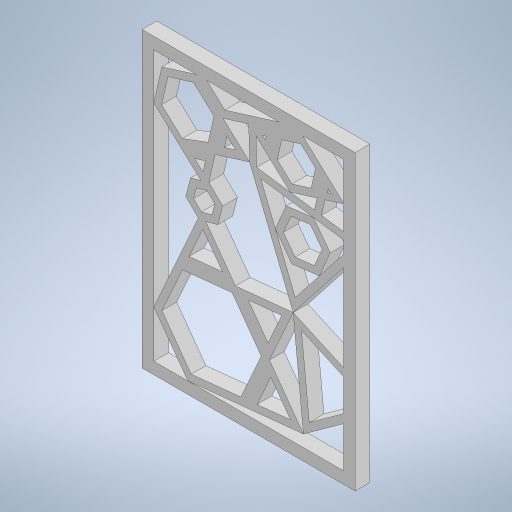
# Autodesk Inventor part: стена
Saved by Autodesk Inventor 2023.1 (Build 271208000, 208)
## iProperties
Created: 2025-12-15
Part Number: стена
Material: Типовые
Document SubType Name: Modeling
Designer: DELL
Density: 1 g/cm^3
Appearance: По умолчанию
Author: DELL
Autodesk Inventor part; units mm, degrees
ref_plane "YZ Plane" through (0, 0, 0) normal (1, 0, 0) x (0, 1, 0)
ref_plane "XZ Plane" through (0, 0, 0) normal (0, 1, 0) x (-1, 0, 0)
ref_plane "XY Plane" through (0, 0, 0) normal (0, 0, 1) x (1, 0, 0)
sketch "Эскиз1" plane through (0, 0, 0) normal (0, 0, 1) x (1, 0, 0)
  line L0 (-18.1641, 25.0477) -> (18.0359, 25.0477)
  line L1 (18.0359, 25.0477) -> (18.0359, -24.7523)
  line L2 (18.0359, -24.7523) -> (-18.1641, -24.7523)
  line L3 (-18.1641, -24.7523) -> (-18.1641, 25.0477)
  line L4 (16.0359, -22.7523) -> (16.0359, 23.0477)
  line L5 (16.0359, 23.0477) -> (-16.1641, 23.0477)
  line L6 (-16.1641, 23.0477) -> (-16.1641, -22.7523)
  line L7 (-16.1641, -22.7523) -> (16.0359, -22.7523)
  line L8 (-10.3906, -22.7523) -> (-16.1641, -14.7523)
  line L9 (-16.1641, -14.7523) -> (-12.1226, -5.7523)
  line L10 (-12.1226, -5.7523) -> (-2.3077, -4.7523)
  line L11 (-2.3077, -4.7523) -> (3.4658, -12.7523)
  line L12 (3.4658, -12.7523) -> (-0.5756, -21.7523)
  line L13 (-0.5756, -21.7523) -> (-10.3906, -22.7523)
  line L14 (-1.3865, -20.6287) -> (2.0873, -12.8928)
  line L15 (2.0873, -12.8928) -> (-2.8753, -6.0164)
  line L16 (-2.8753, -6.0164) -> (-11.3118, -6.8759)
  line L17 (-11.3118, -6.8759) -> (-14.7856, -14.6119)
  line L18 (-14.7856, -14.6119) -> (-9.823, -21.4883)
  line L19 (-9.823, -21.4883) -> (-1.3865, -20.6287)
  line L20 (-0.5756, -21.7523) -> (9.2393, -20.7523)
  line L21 (9.2393, -20.7523) -> (3.4658, -12.7523)
  line L22 (7.0499, -19.7692) -> (1.3705, -20.3478)
  line L23 (3.7091, -15.14) -> (1.3705, -20.3478)
  line L24 (3.7091, -15.14) -> (7.0499, -19.7692)
  line L25 (-12.1226, -5.7523) -> (-8.0812, 3.2477)
  line L26 (-8.0812, 3.2477) -> (-2.3077, -4.7523)
  line L27 (-2.3077, -4.7523) -> (-12.1226, -5.7523)
  line L28 (-10.1765, -4.3478) -> (-4.4971, -3.7692)
  line L29 (-4.4971, -3.7692) -> (-7.8379, 0.86)
  line L30 (-7.8379, 0.86) -> (-10.1765, -4.3478)
  line L31 (3.4658, -12.7523) -> (-2.3077, -4.7523)
  line L32 (-2.3077, -4.7523) -> (7.5073, -3.7523)
  line L33 (7.5073, -3.7523) -> (3.4658, -12.7523)
  line L34 (-0.1183, -5.7355) -> (5.5611, -5.1568)
  line L35 (5.5611, -5.1568) -> (3.2226, -10.3647)
  line L36 (-0.1183, -5.7355) -> (3.2226, -10.3647)
  line L37 (-11.6503, 11.0477) -> (-16.1641, 15.2295)
  line L38 (-16.1641, 15.2295) -> (-14.7994, 21.2295)
  line L39 (-14.7994, 21.2295) -> (-8.9209, 23.0477)
  line L40 (-8.9209, 23.0477) -> (-4.4071, 18.8658)
  line L41 (-4.4071, 18.8658) -> (-5.7718, 12.8658)
  line L42 (-7.1851, 12.4287) -> (-10.4106, 11.4311)
  line L43 (-9.4452, 21.6294) -> (-13.783, 20.2878)
  line L44 (-13.783, 20.2878) -> (-14.8403, 15.6389)
  line L45 (-14.8403, 15.6389) -> (-11.3471, 12.4027)
  line L46 (-11.3471, 12.4027) -> (-6.9303, 14.0695)
  line L47 (-6.9303, 14.0695) -> (-5.9478, 18.3893)
  line L48 (-5.9478, 18.3893) -> (-9.4452, 21.6294)
  line L49 (-5.7718, 12.8658) -> (-7.1365, 6.8658)
  line L50 (-7.1365, 6.8658) -> (-11.6503, 11.0477)
  line L51 (-10.4106, 11.4311) -> (-7.1851, 12.4287)
  line L52 (-7.4029, 11.1053) -> (-7.8262, 9.2438)
  line L53 (-7.8262, 9.2438) -> (-9.2237, 10.5421)
  line L54 (-5.7718, 12.8658) -> (-4.4071, 18.8658)
  line L55 (-4.4071, 18.8658) -> (0.1067, 14.684)
  line L56 (0.1067, 14.684) -> (-5.7718, 12.8658)
  line L57 (-2.2854, 15.2681) -> (-4.1564, 14.6894)
  line L58 (-3.7221, 16.5991) -> (-2.2854, 15.2681)
  line L59 (-3.7221, 16.5991) -> (-4.1564, 14.6894)
  line L60 (-7.4029, 11.1053) -> (-9.2237, 10.5421)
  line L61 (-5.7718, 12.8658) -> (-7.1851, 12.4287)
  line L62 (-10.4106, 11.4311) -> (-11.6503, 11.0477)
  line L63 (7.5073, -3.7523) -> (0.1067, 14.684)
  line L64 (16.0359, 7.1134) -> (7.5073, -3.7523)
  line L65 (16.0359, 9.0569) -> (7.8466, -1.3764)
  line L66 (1.9946, 13.2022) -> (16.0359, 11.1966)
  line L67 (7.8466, -1.3764) -> (1.9946, 13.2022)
  line L68 (0.1067, 14.684) -> (16.0359, 12.4088)
  line L69 (11.9413, 3.8402) -> (7.2772, 3.2858)
  line L70 (7.2772, 3.2858) -> (4.465, 7.0478)
  line L71 (4.465, 7.0478) -> (6.3169, 11.3642)
  line L72 (6.3169, 11.3642) -> (10.981, 11.9186)
  line L73 (10.981, 11.9186) -> (13.7931, 8.1566)
  line L74 (13.7931, 8.1566) -> (11.9413, 3.8402)
  line L75 (7.8235, 4.5592) -> (11.1116, 4.9501)
  line L76 (11.1116, 4.9501) -> (12.4172, 7.9931)
  line L77 (12.4172, 7.9931) -> (10.4346, 10.6452)
  line L78 (10.4346, 10.6452) -> (7.1465, 10.2543)
  line L79 (7.1465, 10.2543) -> (5.841, 7.2113)
  line L80 (5.841, 7.2113) -> (7.8235, 4.5592)
  line L81 (7.5073, -3.7523) -> (9.2393, -20.7523)
  line L82 (9.2393, -20.7523) -> (16.0359, -15.8473)
  line L83 (7.5073, -3.7523) -> (16.0359, -7.5821)
  line L84 (8.9118, -5.6985) -> (16.0359, -8.8976)
  line L85 (10.2225, -18.5629) -> (16.0359, -14.3675)
  line L86 (8.9118, -5.6985) -> (10.2225, -18.5629)
  line L87 (-4.4071, 18.8658) -> (9.1135, 23.0477)
  line L88 (-4.0998, 20.217) -> (5.0524, 23.0477)
  line L89 (-4.0998, 20.217) -> (-7.1552, 23.0477)
  line L90 (6.9877, 13.7011) -> (3.472, 16.9583)
  line L91 (3.472, 16.9583) -> (4.5349, 21.6315)
  line L92 (4.5349, 21.6315) -> (9.1135, 23.0477)
  line L93 (9.1135, 23.0477) -> (12.6293, 19.7905)
  line L94 (12.6293, 19.7905) -> (11.5663, 15.1173)
  line L95 (11.5663, 15.1173) -> (6.9877, 13.7011)
  line L96 (11.3055, 19.3811) -> (8.8062, 21.6965)
  line L97 (8.8062, 21.6965) -> (5.5514, 20.6898)
  line L98 (5.5514, 20.6898) -> (4.7958, 17.3677)
  line L99 (4.7958, 17.3677) -> (7.295, 15.0523)
  line L100 (7.295, 15.0523) -> (10.5499, 16.059)
  line L101 (10.5499, 16.059) -> (11.3055, 19.3811)
  line L102 (11.5663, 15.1173) -> (12.6293, 19.7905)
  line L103 (12.6293, 19.7905) -> (16.0359, 16.6344)
  line L104 (16.145, 16.5334) -> (16.0359, 16.4997) construction
  line L105 (16.0359, 16.6344) -> (16.145, 16.5334) construction
  line L106 (13.4535, 17.3911) -> (13.9482, 16.9327)
  line L107 (13.9482, 16.9327) -> (13.3039, 16.7334)
  line L108 (13.4535, 17.3911) -> (13.3039, 16.7334)
  line L109 (16.0359, 16.4997) -> (11.5663, 15.1173)
  line L110 (12.6293, 19.7905) -> (11.1103, 13.1123)
  line L111 (4.5349, 21.6315) -> (3.472, 16.9583)
  line L112 (3.472, 16.9583) -> (-0.0437, 20.2154)
  line L113 (-0.0437, 20.2154) -> (4.5349, 21.6315)
  line L114 (6.9877, 13.7011) -> (11.1103, 13.1123)
  line L115 (-0.0437, 20.2154) -> (0.1067, 14.684)
  line L116 (1.1878, 19.0745) -> (1.3118, 14.5119)
  line L117 (2.2965, 19.6831) -> (2.9039, 19.871)
  line L118 (2.7629, 19.2511) -> (2.2965, 19.6831)
  line L119 (2.7629, 19.2511) -> (2.9039, 19.871)
  line L120 (12.3023, 12.942) -> (12.8901, 15.5267)
  line L121 (-8.0812, 3.2477) -> (-9.4117, 4.5613)
  line L122 (-9.4117, 4.5613) -> (-8.9393, 6.3704)
  line L123 (-8.9393, 6.3704) -> (-7.1365, 6.8658)
  line L124 (-7.1365, 6.8658) -> (-5.8059, 5.5522)
  line L125 (-5.8059, 5.5522) -> (-6.2783, 3.7431)
  line L126 (-6.2783, 3.7431) -> (-8.0812, 3.2477)
  line L127 (-6.8232, 8.2429) -> (-4.4698, 5.9194)
  line L128 (-4.4698, 5.9194) -> (-5.2923, 2.7696)
  line L129 (-5.2923, 2.7696) -> (-7.3317, 2.2091)
  line L130 (-8.1724, 7.8256) -> (-9.9254, 7.3439)
  line L131 (-9.9254, 7.3439) -> (-10.7478, 4.1941)
  line L132 (-10.7478, 4.1941) -> (-8.6058, 2.0793)
  point P0 (0, 0)
  point P1 (-6.3491, -13.7523)
  point P2 (-7.5038, -2.419)
  point P3 (2.8885, -7.0857)
  point P4 (-10.2856, 17.0477)
  point P5 (-8.1862, 10.2598)
  point P6 (-3.3574, 15.4719)
  point P7 (9.1291, 7.6022)
  point P8 (9.1291, 7.6022)
  point P9 (8.0506, 18.3744)
  point P10 (13.4469, 17.1471)
  point P11 (2.6544, 19.6017)
  point P12 (-7.6088, 5.0568)
  dimension "d0" = 36.2
  dimension "d1" = 49.8
  dimension "d21" = 2
  dimension "d22" = 1.2
  dimension "d24" = 8
  dimension "d25" = 9
  dimension "d26" = 60
  dimension "d27" = 60
  dimension "d31" = 1.2
  dimension "d32" = 1.2
  dimension "d33" = 1.2
  dimension "d39" = 1.2
  dimension "d40" = 1.2
  dimension "d41" = 1.2
  dimension "d44" = 1.2
  dimension "d45" = 1.2
  dimension "d46" = 1.2
  dimension "d47" = 6
  dimension "d48" = 1.2
  dimension "d49" = 1.2
  dimension "d53" = 1.2
  dimension "d74" = 1.2
  dimension "d75" = 60
  dimension "d76" = 60
  dimension "d77" = 1.2
  dimension "d79" = 1.2
  dimension "d81" = 1.2
  dimension "d83" = 1.2
  dimension "d84" = 1.2
  dimension "d85" = 1.2
  dimension "d86" = 60
  dimension "d87" = 60
  dimension "d88" = 60
  dimension "d89" = 1.2
  dimension "d90" = 1.2
  dimension "d100" = 1.2
  dimension "d102" = 1.2
  dimension "d109" = 1.2
  dimension "d113" = 1.2
  dimension "d117" = 1.2
  dimension "d118" = 1.2
  constraints: 264 end point, 19 parallel, 19 point on line, 2 collinear, 2 horizontal, 1 coincident, 1 midpoint, 1 perpendicular, 1 vertical, 148 other
  measures "d0" distance of L1.end L2.end
  measures "d1" distance of L0.end L1.end
  measures "d22" distance between parallel lines of L12 L14
  measures "d24" distance of L8.end L6.end
  measures "d25" vertical distance of L11.end L12.end
  measures "d26" angle of L12 L21
  measures "d27" angle of L12 L20
  measures "d31" distance between parallel lines of L21 L24
  measures "d32" distance between parallel lines of L20 L22
  measures "d33" distance between parallel lines of L12 L23
  measures "d39" distance between parallel lines of L26 L29
  measures "d40" distance between parallel lines of L25 L30
  measures "d41" distance between parallel lines of L10 L28
  measures "d44" distance between parallel lines of L32 L34
  measures "d45" distance between parallel lines of L33 L35
  measures "d46" distance between parallel lines of L11 L36
  measures "d47" vertical distance of L40.end L41.end
  measures "d48" distance between parallel lines of L39 L43
  measures "d49" distance between parallel lines of L49 L52
  measures "d53" distance between parallel lines of L42 L60
  measures "d74" distance between parallel lines of L69 L75
  measures "d75" angle of L81 L82
  measures "d76" angle of L81 L83
  measures "d77" distance between parallel lines of L83 L84
  measures "d79" distance between parallel lines of L82 L85
  measures "d81" distance between parallel lines of L81 L86
  measures "d83" distance between parallel lines of L64 L65
  measures "d84" distance between parallel lines of L63 L67
  measures "d85" distance between parallel lines of L66 L68
  measures "d86" angle of L64 L68
  measures "d87" angle of L63 L68
  measures "d88" angle of L55 L87
  measures "d89" distance between parallel lines of L87 L88
  measures "d90" distance between parallel lines of L40 L89
  measures "d100" distance between parallel lines of L93 L96
  measures "d102" distance between parallel lines of L103 L106
  measures "d109" distance between parallel lines of L115 L116
  measures "d113" distance between parallel lines of L110 L120
  measures "d117" distance between parallel lines of L124 L127
  measures "d118" distance between parallel lines of L123 L130
extrude "Выдавливание1" add sketch "Эскиз1" along normal blind 2.5 contours L0 L1 L2 L3 | L82 L81 L83 L4 L84 L86 L85 | L8 L9 L10 L11 L12 L13 | L20 L12 L21 | L11 L32 L33 | L63 L68 L4 L66 L67 L65 L64 | L38 L39 L40 L41 L61 L42 L62 L37 | L25 L26 L10 | L56 L41 L55 | L115 L112 L116 L68 | L62 L42 L61 L49 L50 | L132 L131 L130 L50 L123 L122 L121 L25 | L26 L126 L125 L124 L49 L127 L128 L129 | L40 L5 L89 L88 L87 | L87 L91 L112 | L90 L91 L87 L93 L94 L95 | L69 L70 L71 L72 L73 L74 | L110 L109 L120 L68 | L94 L103 L4 L109
